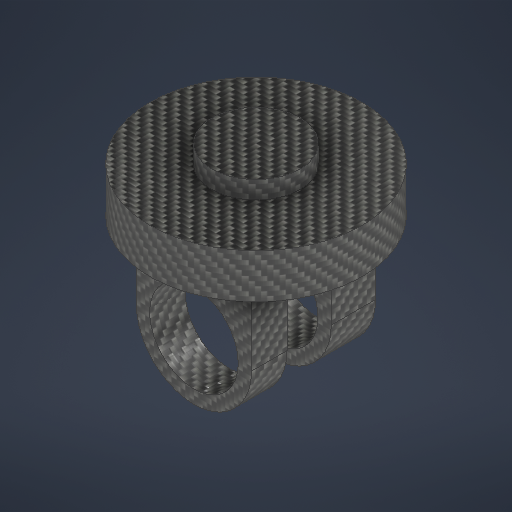
# Autodesk Inventor part: JOINT BASE1
Saved by Autodesk Inventor 2027.1 (Build 311270010, 270A)
## iProperties
Created: 2026-08-28
Part Number: JOINT BASE1
Material: Generic
Document SubType Name: Modeling
Designer: RIDDHIMAN
Density: 1 g/cm^3
Appearance: Default
Author: RIDDHIMAN
Autodesk Inventor part; units mm, degrees
ref_plane "YZ Plane" through (0, 0, 0) normal (1, 0, 0) x (0, 1, 0)
ref_plane "XZ Plane" through (0, 0, 0) normal (0, 1, 0) x (-1, 0, 0)
ref_plane "XY Plane" through (0, 0, 0) normal (0, 0, 1) x (1, 0, 0)
sketch "Sketch1" plane through (0, 0, 0) normal (0, 1, 0) x (-1, 0, 0)
  circle A0 centre (0, 0) radius 60
  dimension "d0" = 120
  constraints: 1 centre point, 1 coincident
  measures "d0" diameter of A0
extrude "Extrusion1" add sketch "Sketch1" along normal mid plane 25
sketch "Sketch2" plane through (0, 12.5, 0) normal (0, 1, 0) x (1, 0, 0)
  circle A0 centre (0, 0) radius 60 projected
  circle A1 centre (0, 0) radius 25
  dimension "d3" = 50
  constraints: 1 centre point, 1 coincident
  measures "d3" diameter of A1
extrude "Extrusion2" add sketch "Sketch2" along normal blind 10 contours A1
sketch "Sketch3" plane through (0, -12.5, 0) normal (0, -1, 0) x (1, 0, 0)
  line L0 (32.5, 35) -> (-32.5, 35)
  line L1 (-32.5, 35) -> (-32.5, -35)
  line L2 (-32.5, -35) -> (32.5, -35)
  line L3 (32.5, -35) -> (32.5, 35)
  line L4 (32.5, 35) -> (-32.5, -35) construction
  line L5 (-32.5, 35) -> (32.5, -35) construction
  line L6 (32.5, 35) -> (-32.5, 35)
  line L7 (-32.5, 35) -> (-32.5, 15)
  line L8 (-32.5, 15) -> (32.5, 15)
  line L9 (32.5, 15) -> (32.5, 35)
  line L10 (32.5, -35) -> (-32.5, -35)
  line L11 (-32.5, -35) -> (-32.5, -10)
  line L12 (-32.5, -10) -> (32.5, -10)
  line L13 (32.5, -10) -> (32.5, -35)
  point P0 (0, 0)
  dimension "d6" = 65
  dimension "d7" = 70
  dimension "d8" = 20
  dimension "d9" = 25
  constraints: 28 end point, 6 parallel, 3 horizontal, 3 perpendicular, 2 midpoint, 2 point on line
  measures "d6" distance of L2.end L1.end
  measures "d7" distance of L1.end L0.end
  measures "d8" distance of L7.end L6.end
  measures "d9" distance of L10.end L11.end
extrude "Extrusion3" add sketch "Sketch3" along normal blind 75 contours L3 L8 L1 L0 | L3 L2 L1 L12
fillet "Fillet1" radius 32.5 4 edges at (32.5, -87.5, 25) (-32.5, -87.5, 25) (-32.5, -87.5, -22.5) (32.5, -87.5, -22.5)
sketch "Sketch4" plane through (-32.5, -12.5, 35) normal (0, 0, 1) x (1, 0, 0)
  circle A0 centre (32.5, -42.5) radius 25
  arc A1 (0, -42.5) -> (65, -42.5) centre (32.5, -42.5) ccw projected
  point P0 (32.5, 12.5)
  dimension "d13" = 50
  constraints: 1 centre point, 1 concentric
  measures "d13" diameter of A0
extrude "Extrusion4" cut sketch "Sketch4" against normal blind 112.75
body "Solid1"
